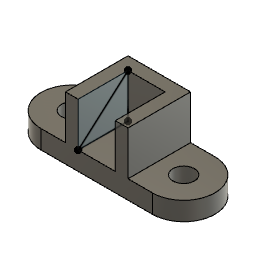
A2 v2 (Autodesk Fusion 360 design; units mm, degrees)
Autodesk Fusion 360 part; units mm, degrees
sketch "Base" plane through (0, 0, 0) normal (0, 1, 0) x (1, 0, 0)
  line L0 (-57, -32) -> (57, -32)
  line L1 (57, 32) -> (-57, 32)
  line L2 (-57, -32) -> (57, 32) construction
  line L3 (57, -32) -> (-57, 32) construction
  circle A0 centre (57, 0) radius 11
  circle A1 centre (-57, 0) radius 11
  arc A2 (-57, 32) -> (-57, -32) centre (-57, 0) ccw
  arc A3 (57, -32) -> (57, 32) centre (57, 0) ccw
  dimension "d1" = 114
  dimension "d2" = 64
  dimension "d3" = 64
  dimension "d4" = 22
  constraint horizontal L0
  constraint parallel L0 L1
  constraint coincident L2 origin
  constraint coincident L3 origin
  constraint concentric A0 A3
  measures "d1" distance of L1.start L1.end
  measures "d2" distance of L0.end L1.start L0.start
  measures "d3" diameter of A3
  measures "d4" diameter of A0
extrude "Extrude1" add sketch "Base" along normal blind 19
sketch "Top piece" plane through (0, 19, 0) normal (0, 1, 0) x (-1, 0, 0)
  circle A0 centre (-57, 0) radius 11
  circle A1 centre (57, 0) radius 11
  arc A2 (-57, 32) -> (-57, -32) centre (-57, 0) ccw
  line L0 (-57, -32) -> (57, -32)
  arc A3 (57, -32) -> (57, 32) centre (57, 0) ccw
  line L1 (57, 32) -> (-57, 32)
  line L2 (-32, 32) -> (32, 32)
  line L3 (32, 32) -> (32, -32)
  line L4 (32, -32) -> (-32, -32)
  line L5 (-32, -32) -> (-32, 32)
  line L6 (-32, 32) -> (32, -32) construction
  line L7 (32, 32) -> (-32, -32) construction
  line L8 (32, 32) -> (19, 32)
  line L9 (19, 32) -> (19, -19)
  line L10 (32, -19) -> (32, 32)
  line L11 (32, -32) -> (-32, -32)
  line L12 (-32, -32) -> (-32, -19)
  line L13 (-19, -19) -> (19, -19)
  line L14 (32, -19) -> (32, -32)
  line L15 (-32, 32) -> (-19, 32)
  line L16 (-19, 32) -> (-19, -19)
  line L17 (-32, -19) -> (-32, 32)
  dimension "d7" = 64
  dimension "d8" = 13
  dimension "d9" = 51
  constraint horizontal L2
  constraint perpendicular L2 L3
  constraint parallel L2 L4
  constraint parallel L3 L5
  constraint coincident L6 origin
  constraint coincident L7 origin
  constraint horizontal L8
  constraint vertical L9
  constraint vertical L10
  constraint horizontal L11
  constraint vertical L12
  constraint horizontal L13
  constraint vertical L14
  constraint coincident L5 L12.end
  constraint horizontal L15
  constraint vertical L16
  constraint vertical L17
  constraint coincident L7 L13.start
  measures "d7" distance of L3.end L4.end
  measures "d8" distance of L2.end L8.end
  measures "d9" distance of L2.end L10.start
extrude "Extrude2" add sketch "Top piece" along normal blind 45 contours L0 L1 L2 L3 L4 L5 L8 L9 L10 L11 L12 L13 L14 L15 L16 L17
sketch "Triangle" plane through (-19, 0, 0) normal (1, 0, 0) x (0, 0, -1)
  line L0 (-32, 19) -> (19, 19)
  line L1 (19, 19) -> (19, 64)
  line L2 (19, 64) -> (-32, 64)
  line L3 (-32, 64) -> (-32, 19)
  line L4 (19, 64) -> (-32, 19)
  line L5 (19, 19) -> (-32, 19)
  line L6 (19, 19) -> (19, 64)
  constraint coincident L1.end L2.start
  constraint coincident L0.start L3.end
  constraint coincident L0.end L1.start
extrude "Extrude3" [suppressed]
named bodies: "Main body"
